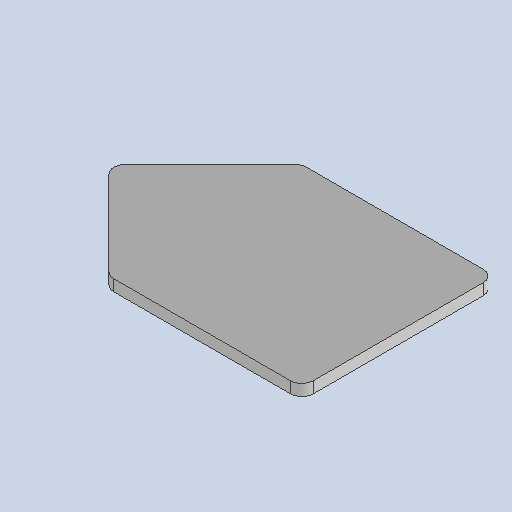
# Autodesk Inventor part: PRS 8666 FDS CUP 1_D940
Saved by Autodesk Inventor 2026.2 (Build 302298000, 298)
## iProperties
Created: 2025-06-24
Part Number: PRS 8666 FDS CUP 1_D940
Material: Stainless Steel
Document SubType Name: Sheet Metal
Designer: admin
Mass: 23.076 g
Surface Area: 31.7918 cm^2
Volume: 2.88451 cm^3
Density: 8 g/cm^3
Flat Pattern Width: 5.01716 cm
Flat Pattern Length: 3.4 cm
Flat Pattern Area: 17.0583 cm^2
Sheet Metal Rule: AISI304 2mm Die16
Sheet Metal Width: 50,172 mm
Sheet Metal Length: 34,000 mm
Sheet Metal Area: 1705,833 mm^2
Appearance: Default
Author: user
Autodesk Inventor part; units mm, degrees
ref_plane "YZ Plane" through (0, 0, 0) normal (1, 0, 0) x (0, 1, 0)
ref_plane "XZ Plane" through (0, 0, 0) normal (0, 1, 0) x (-1, 0, 0)
ref_plane "XY Plane" through (0, 0, 0) normal (0, 0, 1) x (1, 0, 0)
sketch "Sketch1" plane through (0, 0, 0) normal (0, 0, 1) x (1, 0, 0)
  line L0 (-17, -17) -> (17, -17)
  line L1 (17, -17) -> (17, 17)
  line L2 (17, 17) -> (-17, 17)
  line L3 (-17, 17) -> (-17, -17)
  line L4 (-17, -17) -> (17, 17) construction
  line L5 (17, -17) -> (-17, 17) construction
  line L6 (-17, -17) -> (-34, 0)
  line L7 (-34, 0) -> (-17, 17)
  point P0 (0, 0)
  point P1 (-17, 0)
  dimension "d154" = 34
  dimension "d155" = 34
  dimension "d180" = 17
  measures "d154" distance of L1.end L2.end
  measures "d155" distance of L0.end L1.end
  measures "d180" distance from line of L6.end L3
extrude "Plate5" add sketch "Sketch1" along normal blind 2
fillet "Corner Round1" radius 2 5 edges at (17, 17, 1) (-17, 17, 1) (-17, -17, 1) (17, -17, 1) (-34, 0, 1)
body "Solid3"
